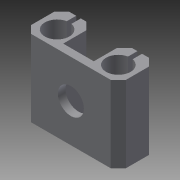
# Autodesk Inventor part: XCarriageV3
Saved by Autodesk Inventor 2015 (Build 190159000, 159)
## iProperties
Created: 2014-08-17
Part Number: XCarriageV3
Material: Generic
Document SubType Name: Modeling
Designer: Jack
Density: 1 g/cm^3
Appearance: Default
Author: Jack
Autodesk Inventor part; units mm, degrees
ref_plane "YZ Plane" through (0, 0, 0) normal (1, 0, 0) x (0, 1, 0)
ref_plane "XZ Plane" through (0, 0, 0) normal (0, 1, 0) x (-1, 0, 0)
ref_plane "XY Plane" through (0, 0, 0) normal (0, 0, 1) x (1, 0, 0)
sketch "Sketch1" plane through (0, 0, 0) normal (0, 0, 1) x (1, 0, 0)
  arc A0 (-1.5, 7.8581) -> (1.5, 7.8581) centre (0, 0) ccw
  arc A1 (38.5, 7.8581) -> (41.5, 7.8581) centre (40, 0) ccw
  line L0 (-1.5, 7.8581) -> (-1.5, 14)
  line L1 (-1.5, 14) -> (-11, 14)
  line L2 (-11, 14) -> (-11, -11)
  line L3 (-11, -11) -> (51, -11)
  line L4 (51, -11) -> (51, 14)
  line L5 (51, 14) -> (41.5, 14)
  line L6 (41.5, 14) -> (41.5, 7.8581)
  line L7 (1.5, 7.8581) -> (1.5, 14)
  line L8 (1.5, 14) -> (10, 14)
  line L9 (10, 14) -> (10, -6)
  line L10 (10, -6) -> (30, -6)
  line L11 (30, -6) -> (30, 14)
  line L12 (30, 14) -> (38.5, 14)
  line L13 (38.5, 14) -> (38.5, 7.8581)
  dimension "d0" = 16
  dimension "d1" = 16
  dimension "d2" = 40
  dimension "d3" = 1.5
  dimension "d4" = 1.5
  dimension "d5" = 1.5
  dimension "d6" = 1.5
  dimension "d7" = 11
  dimension "d8" = 10
  dimension "d9" = 14
  dimension "d10" = 10
  dimension "d11" = 11
  dimension "d12" = 11
  dimension "d13" = 5
  constraints: 28 end point, 10 perpendicular, 4 point on circle, 4 point on line, 2 centre point, 2 horizontal alignment, 2 vertical, 1 coincident
  measures "d0" diameter of A0
  measures "d1" diameter of A1
  measures "d2" distance of A1.centre point (0, 0)
  measures "d3" distance from line of L13 A1.centre
  measures "d4" distance from line of A1.centre L6
  measures "d5" distance from line of point (0, 0) L7
  measures "d6" distance from line of point (0, 0) L0
  measures "d7" distance from line of point (0, 0) L2
  measures "d8" distance from line of L9 point (0, 0)
  measures "d9" distance from line of point (0, 0) L8
  measures "d10" distance from line of A1.centre L11
  measures "d11" distance from line of L4 A1.centre
  measures "d12" distance from line of L3 point (0, 0)
  measures "d13" distance between parallel lines of L3 L10
extrude "Extrusion1" add sketch "Sketch1" along normal blind 50
sketch "Sketch2" plane through (10, -6, 0) normal (0, 1, 0) x (1, 0, 0)
  line L0 (0, 0) -> (20, 0) projected
  line L1 (20, 0) -> (20, -50) projected
  circle A0 centre (10, -25) radius 8.5
  point P0 (-10, 0)
  dimension "d16" = 17
  dimension "d17" = 10
  dimension "d18" = 25
  constraints: 1 centre point
  measures "d16" diameter of A0
  measures "d17" distance from line of L1 A0.centre
  measures "d18" distance from line of L0 A0.centre
extrude "Extrusion2" cut sketch "Sketch2" against normal up to surface (5 mm away)
chamfer "Chamfer1" distance 5 angle 45 4 edges at (-11, 14, 25) (10, 14, 25) (30, 14, 25) (51, 14, 25)
chamfer "Chamfer2" distance 5 angle 45 2 edges at (-11, -11, 25) (51, -11, 25)
body "Solid1"
